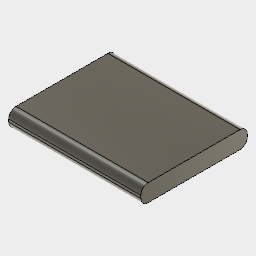
1578 500mAh battery (Autodesk Fusion 360 design; units mm, degrees)
Autodesk Fusion 360 part; units mm, degrees
sketch "Sketch1" plane through (0, 0, 0) normal (0, 0, 1) x (1, 0, 0)
  line L0 (0, 0) -> (36, 0)
  line L1 (36, 0) -> (36, 29)
  line L2 (36, 29) -> (0, 29)
  line L3 (0, 29) -> (0, 0)
  dimension "d1" = 36
  dimension "d2" = 29
  measures "d1" distance of L1.end L2.end
  measures "d2" distance of L0.start L2.end
extrude "Extrude1" add sketch "Sketch1" along normal blind 4.75
fillet "Fillet1" radius 2 4 edges at (18, 0, 4.75) (18, 0, 0) (18, 29, 4.75) (18, 29, 0)
